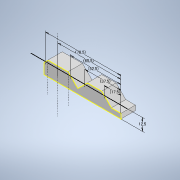
# Autodesk Inventor part: finger2
Saved by Autodesk Inventor 2021 (Build 250183000, 183)
## iProperties
Created: 2021-12-29
Part Number: finger2
Material: 一般
Document SubType Name: Modeling
Designer: shibu
Density: 1 g/cm^3
Appearance: 既定
Author: shibu
Autodesk Inventor part; units mm, degrees
ref_plane "YZ Plane" through (0, 0, 0) normal (1, 0, 0) x (0, 1, 0)
ref_plane "XZ Plane" through (0, 0, 0) normal (0, 1, 0) x (-1, 0, 0)
ref_plane "XY Plane" through (0, 0, 0) normal (0, 0, 1) x (1, 0, 0)
sketch "スケッチ3" plane through (0, 0, 0) normal (0, 0, 1) x (1, 0, 0)
  line L0 (0, 0) -> (0, 5)
  line L1 (0, 5) -> (-10, 5)
  line L2 (-10, 5) -> (-20, 15)
  line L3 (-20, 15) -> (-35, 15)
  line L4 (-35, 15) -> (-45, 5)
  line L5 (-45, 5) -> (-55, 15)
  line L6 (-80, 0) -> (0, 0)
  line L7 (0, 5) -> (0, 0)
  line L8 (-55, 15) -> (-80, 15)
  line L9 (-80, 15) -> (-80, 0)
  dimension "d0" = 10
  dimension "d2" = 15
  dimension "d4" = 5
  dimension "d6" = 135
  dimension "d9" = 25
  dimension "d10" = 15
  constraints: 20 end point, 4 perpendicular, 2 parallel, 2 point on line, 1 horizontal, 1 vertical
  measures "d0" distance of L0.end L1.end
  measures "d2" distance of L2.end L3.end
  measures "d4" distance between parallel lines of L6 L1
  measures "d6" angle of L2 L1
  measures "d9" distance from line of L9 L5.end
  measures "d10" distance between parallel lines of L6 L8
extrude "押し出し1" add sketch "スケッチ3" along normal blind 15
chamfer "面取り1" distance 4 angle 45 1 edges at (-80, 15, 7.5)
sketch "スケッチ4" plane through (0, 0, 15) normal (0, 0, 1) x (1, 0, 0)
  line L0 (-80, 11) -> (-76, 15) projected
  line L1 (-80, 11) -> (-80, 0) projected
  line L2 (-80, 0) -> (0, 0) projected
  line L3 (0, 0) -> (0, 5) projected
  line L4 (0, 5) -> (-10, 5) projected
  line L5 (-10, 5) -> (-20, 15) projected
  line L6 (-20, 15) -> (-35, 15) projected
  line L7 (-35, 15) -> (-45, 5) projected
  line L8 (-45, 5) -> (-55, 15) projected
  line L9 (-55, 15) -> (-76, 15) projected
  line L10 (-93.9194, 12.5) -> (6.2827, 12.5)
  line L11 (-45, 5) -> (-55, 15) projected
  line L12 (-35, 15) -> (-45, 5) projected
  line L13 (-10, 5) -> (-20, 15) projected
  line L14 (-65.5, 45.5) -> (-65.5, -30.5) construction
  line L15 (-55, 15) -> (-76, 15) construction
  line L16 (-55, 15) -> (-55, -16.6145) construction
  line L17 (-76, 15) -> (-76, -16.6145) construction
  point P0 (-78.5, 12.5)
  point P1 (-52.5, 12.5)
  point P2 (-37.5, 12.5)
  point P3 (-17.5, 12.5)
  dimension "d14" = 12.5
  dimension "d15" = 17.5
  dimension "d16" = 37.5
  dimension "d17" = 52.5
  dimension "d18" = 78.5
  dimension "d19" = 65.5
  constraints: 8 end point, 8 point on line, 3 vertical, 1 horizontal, 1 other
  measures "d14" distance between parallel lines of L10 L2
  measures "d15" distance from line of L3 point (-17.5, 12.5)
  measures "d16" distance from line of point (-37.5, 12.5) L3
  measures "d17" distance from line of point (-52.5, 12.5) L3
  measures "d18" distance from line of point (-78.5, 12.5) L3
  measures "d19" distance between parallel lines of L3 L14
